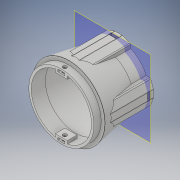
# Autodesk Inventor part: endkappen_V4
Saved by Autodesk Inventor 2017 (Build 210142000, 142)
## iProperties
Part Number: endkappen_V4
Material: Generisch
Document SubType Name: Modeling
Designer: Fabio
Density: 1 g/cm^3
Appearance: Vorgabe
Author: Fabio
Autodesk Inventor part; units mm, degrees
ref_plane "YZ Plane" through (0, 0, 0) normal (1, 0, 0) x (0, 1, 0)
ref_plane "XZ Plane" through (0, 0, 0) normal (0, 1, 0) x (-1, 0, 0)
ref_plane "XY Plane" through (0, 0, 0) normal (0, 0, 1) x (1, 0, 0)
sketch "Skizze2" plane through (0, 0, 0) normal (1, 0, 0) x (0, 1, 0)
  line L0 (0, 0) -> (48.6481, 0)
  line L1 (47.4748, 20) -> (47.4748, 25)
  line L2 (6, 30) -> (6, 27)
  line L3 (6, 27) -> (0, 27)
  line L4 (6.2626, 30) -> (6, 30)
  line L5 (11.7576, 25) -> (0, 25)
  line L6 (0, 25) -> (0, 27)
  line L7 (0, 0) -> (0, 25) construction
  line L8 (40.5337, 20) -> (47.4748, 20)
  line L9 (11.7576, 25) -> (40.5337, 20)
  line L10 (47.4748, 25) -> (35.0388, 25)
  line L11 (6.2626, 30) -> (35.0388, 25)
  dimension "d164" = 60
  dimension "d166" = 54
  dimension "d167" = 50
  dimension "d168" = 6
  dimension "d171" = 47.4748
  dimension "d174" = 40.5337
  dimension "d203" = 3
  dimension "d204" = 40
  dimension "d205" = 5
  dimension "d206" = 170.143
  dimension "d207" = 12.436
  constraints: 24 end point, 5 horizontal, 2 vertical, 1 parallel, 1 perpendicular
  measures "d164" diameter of L4 L0
  measures "d166" diameter of L3 L0
  measures "d167" diameter of L5 L0
  measures "d168" distance of L2.end L3.end
  measures "d171" distance of L5.end L1.end
  measures "d174" distance from line of L7 L8.start
  measures "d203" distance of L2.start L2.end
  measures "d204" diameter of L8 L0
  measures "d205" distance of L1.start L1.end
  measures "d206" angle of L5 L9
  measures "d207" distance of L1.end L10.end
revolve "Umdrehung1" add sketch "Skizze2" angle 360 about axis through (0, 0, 0) along (0, 1, 0)
sketch "Skizze18" plane through (0, 0, 0) normal (0, -1, 0) x (1, 0, 0)
  circle A0 centre (0, 0) radius 25 projected
  line L0 (5, -22) -> (-5, -22)
  line L1 (-5, -22) -> (-5, -25)
  line L2 (-5, -25) -> (5, -25)
  line L3 (5, -25) -> (5, -22)
  line L4 (5, -22) -> (-5, -25) construction
  line L5 (-5, -22) -> (5, -25) construction
  line L6 (0, -23.5) -> (0, 0) construction
  line L7 (0, 0) -> (9.0804, 0) construction
  line L8 (5, 22) -> (-5, 22)
  line L9 (-5, 22) -> (-5, 25)
  line L10 (-5, 25) -> (5, 25)
  line L11 (5, 25) -> (5, 22)
  dimension "d176" = 10
  dimension "d177" = 3
  dimension "d178" = 22
  constraints: 24 end point, 4 symmetric about line, 2 horizontal, 2 midpoint, 2 parallel, 1 perpendicular, 1 vertical
  measures "d176" distance of L2.end L1.end
  measures "d177" distance of L0.end L1.end
  measures "d178" distance from line of point (0, 0) L0
extrude "Extrusion14" add sketch "Skizze18" against normal blind 8 contours L11 L8 L9 A0 | A0 L10 L11 | L3 L2 A0 | A0 L1 L0 L3 | A0 L9 L10 | L2 L1 A0
sketch "Skizze19" plane through (0, 0, 0) normal (0, -1, 0) x (1, 0, 0)
  arc A0 (-5, -24.4949) -> (5, -24.4949) centre (0, 0) ccw projected
  line L0 (0, 0) -> (9.7237, 0) construction
  line L1 (0, -24.5) -> (0, 0) construction
  line L2 (2.85, -23.5) -> (-2.85, -23.5)
  line L3 (-2.85, -23.5) -> (-2.85, -25.5)
  line L4 (-2.85, -25.5) -> (2.85, -25.5)
  line L5 (2.85, -25.5) -> (2.85, -23.5)
  line L6 (2.85, -23.5) -> (-2.85, -25.5) construction
  line L7 (-2.85, -23.5) -> (2.85, -25.5) construction
  line L8 (2.85, 23.5) -> (-2.85, 23.5)
  line L9 (-2.85, 23.5) -> (-2.85, 25.5)
  line L10 (-2.85, 25.5) -> (2.85, 25.5)
  line L11 (2.85, 25.5) -> (2.85, 23.5)
  dimension "d236" = 5.7
  dimension "d237" = 2
  dimension "d238" = 23.5
  constraints: 24 end point, 4 symmetric about line, 2 horizontal, 2 midpoint, 2 parallel, 1 perpendicular, 1 vertical
  measures "d236" distance of L4.end L3.end
  measures "d237" distance of L3.end L2.end
  measures "d238" distance between parallel lines of L0 L2
extrude "Extrusion15" cut sketch "Skizze19" against normal blind 5.7
sketch "Skizze20" plane through (5, 0, 22) normal (0, 0, -1) x (-1, 0, 0)
  line L0 (10, 0) -> (0, 0) projected
  line L1 (10, 0) -> (10, 8) projected
  point P0 (5, 0)
  point P1 (5, 2.85)
  dimension "d185" = 2.85
  dimension "d186" = 5
  measures "d185" distance from line of L0 point (5, 2.85)
  measures "d186" distance from line of L1 point (5, 2.85)
hole "Bohrung4" at (0, 2.85, 22) direction (0, 0, 1) diameter 3.3 end through all
sketch "Skizze21" plane through (-5, 0, -22) normal (0, 0, 1) x (1, 0, 0)
  line L0 (10, 0) -> (0, 0) projected
  line L1 (0, 0) -> (0, 8) projected
  point P0 (5, 0)
  point P1 (5, 2.85)
  dimension "d194" = 2.85
  dimension "d195" = 5
  measures "d194" distance from line of point (5, 2.85) L0
  measures "d195" distance from line of L1 point (5, 2.85)
hole "Bohrung5" at (0, 2.85, -22) direction (0, 0, -1) diameter 3.3 end through all
sketch "Skizze38" plane through (0, 47.4748, 0) normal (0, 1, 0) x (1, 0, 0)
  circle A0 centre (0, 0) radius 25 projected
  line L0 (-10, -25.7127) -> (-10, -22.9129)
  line L1 (-10, -22.9129) -> (10, -22.9129)
  line L2 (10, -22.9129) -> (10, -25.6895)
  circle A1 centre (0, 0) radius 27 projected
  line L3 (-2.955, -28.9129) -> (2.8913, -28.9129)
  line L4 (3.2333, -28.8526) -> (9.342, -26.6292)
  line L5 (-3.297, -28.8526) -> (-9.342, -26.6524)
  arc A2 (2.8913, -28.9129) -> (3.2333, -28.8526) centre (2.8913, -27.9129) ccw
  arc A3 (-3.297, -28.8526) -> (-2.955, -28.9129) centre (-2.955, -27.9129) ccw
  arc A4 (-10, -25.7127) -> (-9.342, -26.6524) centre (-9, -25.7127) ccw
  arc A5 (9.342, -26.6292) -> (10, -25.6895) centre (9, -25.6895) ccw
  arc A6 (28.8526, -3.297) -> (28.9129, -2.955) centre (27.9129, -2.955) ccw
  line L6 (28.8526, -3.297) -> (26.6524, -9.342)
  arc A7 (25.7127, -10) -> (26.6524, -9.342) centre (25.7127, -9) ccw
  line L7 (25.7127, -10) -> (22.9129, -10)
  line L8 (28.9129, -2.955) -> (28.9129, 2.8913)
  line L9 (22.9129, -10) -> (22.9129, 10)
  arc A8 (28.9129, 2.8913) -> (28.8526, 3.2333) centre (27.9129, 2.8913) ccw
  line L10 (22.9129, 10) -> (25.6895, 10)
  arc A9 (26.6292, 9.342) -> (25.6895, 10) centre (25.6895, 9) ccw
  line L11 (28.8526, 3.2333) -> (26.6292, 9.342)
  arc A10 (3.297, 28.8526) -> (2.955, 28.9129) centre (2.955, 27.9129) ccw
  line L12 (3.297, 28.8526) -> (9.342, 26.6524)
  arc A11 (10, 25.7127) -> (9.342, 26.6524) centre (9, 25.7127) ccw
  line L13 (10, 25.7127) -> (10, 22.9129)
  line L14 (2.955, 28.9129) -> (-2.8913, 28.9129)
  line L15 (10, 22.9129) -> (-10, 22.9129)
  arc A12 (-2.8913, 28.9129) -> (-3.2333, 28.8526) centre (-2.8913, 27.9129) ccw
  line L16 (-10, 22.9129) -> (-10, 25.6895)
  arc A13 (-9.342, 26.6292) -> (-10, 25.6895) centre (-9, 25.6895) ccw
  line L17 (-3.2333, 28.8526) -> (-9.342, 26.6292)
  arc A14 (-28.8526, 3.297) -> (-28.9129, 2.955) centre (-27.9129, 2.955) ccw
  line L18 (-28.8526, 3.297) -> (-26.6524, 9.342)
  arc A15 (-25.7127, 10) -> (-26.6524, 9.342) centre (-25.7127, 9) ccw
  line L19 (-25.7127, 10) -> (-22.9129, 10)
  line L20 (-28.9129, 2.955) -> (-28.9129, -2.8913)
  line L21 (-22.9129, 10) -> (-22.9129, -10)
  arc A16 (-28.9129, -2.8913) -> (-28.8526, -3.2333) centre (-27.9129, -2.8913) ccw
  line L22 (-22.9129, -10) -> (-25.6895, -10)
  arc A17 (-26.6292, -9.342) -> (-25.6895, -10) centre (-25.6895, -9) ccw
  line L23 (-28.8526, -3.2333) -> (-26.6292, -9.342)
  point P0 (-10, -26.4129)
  point P1 (-3.1313, -28.9129)
  point P2 (3.0676, -28.9129)
  point P3 (28.9129, -3.1313)
  point P4 (26.4129, -10)
  point P5 (28.9129, 3.0676)
  point P6 (3.1313, 28.9129)
  point P7 (10, 26.4129)
  point P8 (-3.0676, 28.9129)
  point P9 (-28.9129, 3.1313)
  point P10 (-26.4129, 10)
  point P11 (-28.9129, -3.0676)
  dimension "d325" = 20
  dimension "d326" = 3.5
  dimension "d329" = 6
  dimension "d330" = 22.9129
  dimension "d331" = 110
  dimension "d332" = 110
  dimension "d333" = 160
  dimension "d336" = 6.1989
  dimension "d337" = 1
  dimension "d340" = 360
  constraints: 48 end point, 32 point on circle, 24 point on line, 16 centre point, 8 tangent, 3 equal radius, 1 horizontal, 1 parallel, 111 other
  measures "d325" distance of L0.end L1.end
  measures "d326" distance of point (-10, -26.413) L0.end
  measures "d329" distance between parallel lines of L1 L3
  measures "d330" distance from line of point (0, 0) L1
  measures "d331" angle of L2 L4
  measures "d332" angle of L5 L0
  measures "d333" angle of L3 L5
  measures "d336" distance of point (-3.131, -28.913) point (3.068, -28.913)
  measures "d337" radius of A2
extrude "Extrusion27" add sketch "Skizze38" against normal blind 37 contours A0 L9 | A0 L10 A1 L7 | L15 A0 | A0 L16 A1 L13 | L10 A9 L11 A8 L8 A6 L6 A7 L7 A1 | L2 A1 L0 A0 | A0 L1 | A1 L16 A13 L17 A12 L14 A10 L12 A11 L13 | L2 A5 L4 A2 L3 A3 L5 A4 L0 A1 | L21 A0 | A0 L22 A1 L19 | A1 L22 A17 L23 A16 L20 A14 L18 A15 L19
sketch "Skizze39" plane through (-2.955, 47.4748, 28.9129) normal (0, 1, 0) x (1, 0, 0)
  line L0 (-7.045, 6) -> (-7.045, 3.2002) projected
  point P0 (2.955, 28.9129)
  point P1 (2.955, 3.4129)
  point P2 (28.455, 28.9129)
  point P3 (2.955, 54.4129)
  point P4 (-22.545, 28.9129)
  dimension "d344" = 25.5
  dimension "d345" = 10
  dimension "d348" = 360
  constraints: 5 other
  measures "d344" distance of point (2.955, 28.913) point (2.955, 3.413)
  measures "d345" distance from line of L0 point (2.955, 3.413)
hole "Bohrung10" at (0, 47.4748, 25.5) at (25.5, 47.4748, 0) at (0, 47.4748, -25.5) at (-25.5, 47.4748, 0) direction (0, -1, 0) diameter 3.3 depth 8 tip angle 118
delete faces "Fläche löschen16" heal yes whole lump no faces at (-2.4824, 12.6428, 22.9129) (-2.2576, 10.4748, 23.2969)
delete faces "Fläche löschen17" heal yes whole lump no faces at (22.9129, 15.7136, -2.6784) (23.4328, 10.4748, 1.7026)
delete faces "Fläche löschen18" heal yes whole lump no faces at (0, 10.4748, -23.6086) (-2.6784, 15.7136, -22.9129)
delete faces "Fläche löschen19" heal yes whole lump no faces at (-23.4328, 10.4748, -1.7026) (-22.9129, 15.7136, 2.6784)
ref_plane "Arbeitsebene6" through (-2.8913, 42.4748, -28.9129) normal (0, 1, 0) x (1, 0, 0)
sketch "Skizze42" plane through (-2.8913, 42.4748, -28.9129) normal (0, 1, 0) x (1, 0, 0)
  circle A0 centre (2.8913, -54.4129) radius 1.65 projected
  line L0 (5.7413, -51.5629) -> (0.0413, -51.5629)
  line L1 (0.0413, -51.5629) -> (0.0413, -57.2629)
  line L2 (0.0413, -57.2629) -> (5.7413, -57.2629)
  line L3 (5.7413, -57.2629) -> (5.7413, -51.5629)
  line L4 (5.7413, -51.5629) -> (0.0413, -57.2629) construction
  line L5 (0.0413, -51.5629) -> (5.7413, -57.2629) construction
  line L6 (25.5413, -26.0629) -> (25.5413, -31.7629)
  line L7 (25.5413, -31.7629) -> (31.2413, -31.7629)
  line L8 (31.2413, -31.7629) -> (31.2413, -26.0629)
  line L9 (31.2413, -26.0629) -> (25.5413, -26.0629)
  line L10 (25.5413, -26.0629) -> (31.2413, -31.7629) construction
  line L11 (25.5413, -31.7629) -> (31.2413, -26.0629) construction
  line L12 (0.0413, -6.2629) -> (5.7413, -6.2629)
  line L13 (5.7413, -6.2629) -> (5.7413, -0.5629)
  line L14 (5.7413, -0.5629) -> (0.0413, -0.5629)
  line L15 (0.0413, -0.5629) -> (0.0413, -6.2629)
  line L16 (0.0413, -6.2629) -> (5.7413, -0.5629) construction
  line L17 (5.7413, -6.2629) -> (0.0413, -0.5629) construction
  line L18 (-19.7587, -31.7629) -> (-19.7587, -26.0629)
  line L19 (-19.7587, -26.0629) -> (-25.4587, -26.0629)
  line L20 (-25.4587, -26.0629) -> (-25.4587, -31.7629)
  line L21 (-25.4587, -31.7629) -> (-19.7587, -31.7629)
  line L22 (-19.7587, -31.7629) -> (-25.4587, -26.0629) construction
  line L23 (-19.7587, -26.0629) -> (-25.4587, -31.7629) construction
  point P0 (2.8913, -28.9129)
  dimension "d358" = 5.7
  dimension "d359" = 5.7
  dimension "d362" = 360
  constraints: 48 end point, 2 midpoint, 2 parallel, 1 horizontal, 1 perpendicular, 41 other
  measures "d358" distance of L2.end L1.end
  measures "d359" distance of L1.end L0.end
extrude "Extrusion28" cut sketch "Skizze42" along normal blind 2 contours A0 | L3 L2 L1 L0 | L9 L8 L7 L6 | L15 L14 L13 L12 | L21 L20 L19 L18
sketch "Skizze43" plane through (-2.8913, 42.4748, -28.9129) normal (0, 1, 0) x (1, 0, 0)
  circle A0 centre (28.3913, -28.9129) radius 1.65 projected
  line L0 (28.3913, -26.0629) -> (32.4585, -26.0629)
  line L1 (32.4585, -26.0629) -> (32.4585, -31.7629)
  line L2 (32.4585, -31.7629) -> (28.3913, -31.7629)
  line L3 (28.3913, -26.0629) -> (28.3913, -31.7629)
  line L4 (32.4585, -26.0629) -> (28.3913, -31.7629) construction
  line L5 (32.4585, -31.7629) -> (28.3913, -26.0629) construction
  line L6 (0.0413, -3.4129) -> (0.0413, 0.6543)
  line L7 (0.0413, 0.6543) -> (5.7413, 0.6543)
  line L8 (5.7413, 0.6543) -> (5.7413, -3.4129)
  line L9 (0.0413, -3.4129) -> (5.7413, -3.4129)
  line L10 (0.0413, 0.6543) -> (5.7413, -3.4129) construction
  line L11 (5.7413, 0.6543) -> (0.0413, -3.4129) construction
  line L12 (-22.6087, -31.7629) -> (-26.6758, -31.7629)
  line L13 (-26.6758, -31.7629) -> (-26.6758, -26.0629)
  line L14 (-26.6758, -26.0629) -> (-22.6087, -26.0629)
  line L15 (-22.6087, -31.7629) -> (-22.6087, -26.0629)
  line L16 (-26.6758, -31.7629) -> (-22.6087, -26.0629) construction
  line L17 (-26.6758, -26.0629) -> (-22.6087, -31.7629) construction
  line L18 (5.7413, -54.4129) -> (5.7413, -58.48)
  line L19 (5.7413, -58.48) -> (0.0413, -58.48)
  line L20 (0.0413, -58.48) -> (0.0413, -54.4129)
  line L21 (5.7413, -54.4129) -> (0.0413, -54.4129)
  line L22 (5.7413, -58.48) -> (0.0413, -54.4129) construction
  line L23 (0.0413, -58.48) -> (5.7413, -54.4129) construction
  point P0 (2.8913, -28.9129)
  dimension "d366" = 5.7
  dimension "d367" = 4.0672
  dimension "d368" = 25.5
  dimension "d369" = 4.0672
  dimension "d370" = 5.7
  dimension "d371" = 2.85
  dimension "d374" = 360
  constraints: 48 end point, 1 horizontal, 1 parallel, 1 perpendicular, 41 other
  measures "d366" distance of L0.end L1.end
  measures "d367" distance of L0.start L0.end
  measures "d368" distance from line of point (2.891, -28.913) L3
  measures "d369" distance of L1.end L2.end
  measures "d370" distance of L0.start L2.end
  measures "d371" distance from line of L2 A0.centre
extrude "Extrusion29" cut sketch "Skizze43" along normal blind 2
